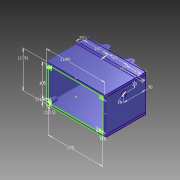
# Autodesk Inventor part: BoxSolidWalls
Saved by Autodesk Inventor 2015 (Build 190159000, 159)
## iProperties
Created: 2015-04-29
Part Number: BoxSolidWalls
Material: ABS Plastic
Document SubType Name: Modeling
Designer: Akovo_000
Mass: 583.352 g
Surface Area: 1681.04 cm^2
Volume: 550.333 cm^3
Density: 1.06 g/cm^3
Appearance: Smooth - White
Author: Akovo_000
Autodesk Inventor part; units mm, degrees
note: some values were not read from the file. Chosen so that the rebuilt part matches the saved one: sketch regions of "LensplateMount".
(part 1 of 2)
ref_plane "YZ Plane" through (0, 0, 0) normal (1, 0, 0) x (0, 1, 0)
ref_plane "XZ Plane" through (0, 0, 0) normal (0, 1, 0) x (-1, 0, 0)
ref_plane "XY Plane" through (0, 0, 0) normal (0, 0, 1) x (1, 0, 0)
sketch "BasicBox" plane through (0, 0, 0) normal (0, 1, 0) x (-1, 0, 0)
  line L0 (88.0422, 45.0444) -> (-86.9578, 45.0444)
  line L1 (-86.9578, 45.0444) -> (-86.9578, -59.9556)
  line L2 (-86.9578, -59.9556) -> (88.0422, -59.9556)
  line L3 (88.0422, -59.9556) -> (88.0422, 45.0444)
  line L4 (95.0422, 52.0444) -> (-93.9578, 52.0444)
  line L5 (-93.9578, 52.0444) -> (-93.9578, -66.9556)
  line L6 (-93.9578, -66.9556) -> (95.0422, -66.9556)
  line L7 (95.0422, -66.9556) -> (95.0422, 52.0444)
  line L8 (88.0422, 45.0444) -> (88.0422, 45.5444) construction
  line L9 (88.0422, 45.0444) -> (88.5422, 45.0444) construction
  line L10 (88.0422, -59.9556) -> (88.0422, -60.4556) construction
  line L11 (88.0422, -59.9556) -> (88.5422, -59.9556) construction
  line L12 (-86.9578, -59.9556) -> (-86.9578, -60.4556) construction
  line L13 (-86.9578, 45.0444) -> (-86.9578, 45.5444) construction
  line L14 (-86.9578, 45.0444) -> (-87.4578, 45.0444) construction
  line L15 (-86.9578, -59.9556) -> (-87.4578, -59.9556) construction
  line L16 (-87.4578, -60.4556) -> (-87.4578, -59.9556)
  line L17 (-87.4578, 45.5444) -> (-86.9578, 45.5444)
  line L18 (88.5422, 45.5444) -> (88.5422, -59.9556)
  line L19 (88.5422, -60.4556) -> (88.0422, -60.4556)
  line L20 (88.5422, 45.0444) -> (95.0422, 45.0444) construction
  line L21 (88.0422, 45.5444) -> (88.0422, 52.0444) construction
  line L22 (-86.9578, 45.5444) -> (88.5422, 45.5444)
  line L23 (-87.4578, 45.0444) -> (-87.4578, 45.5444)
  line L24 (-87.4578, -59.9556) -> (-87.4578, 45.0444)
  line L25 (-86.9578, -60.4556) -> (-87.4578, -60.4556)
  line L26 (88.5422, -59.9556) -> (88.5422, -60.4556)
  line L27 (88.0422, -60.4556) -> (-86.9578, -60.4556)
  line L28 (88.5422, -59.9556) -> (95.0422, -59.9556) construction
  line L29 (88.0422, -60.4556) -> (88.0422, -66.9556) construction
  line L30 (-87.4578, 45.0444) -> (-93.9578, 45.0444) construction
  line L31 (-86.9578, 45.5444) -> (-86.9578, 52.0444) construction
  line L32 (-87.4578, -59.9556) -> (-93.9578, -59.9556) construction
  line L33 (-86.9578, -60.4556) -> (-86.9578, -66.9556) construction
  line L34 (-76.9578, -59.9556) -> (-76.9578, -49.9556)
  line L35 (-76.9578, -49.9556) -> (-86.9578, -49.9556)
  line L36 (-76.9578, 45.0444) -> (-76.9578, 35.0444)
  line L37 (-76.9578, 35.0444) -> (-86.9578, 35.0444)
  line L38 (78.5422, 45.0444) -> (78.5422, 35.0444)
  line L39 (78.5422, 35.0444) -> (88.0422, 35.0444)
  line L40 (88.5422, -49.9556) -> (78.5422, -49.9556)
  line L41 (78.5422, -49.9556) -> (78.5422, -59.9556)
  line L42 (78.5422, 45.0444) -> (78.5422, 52.0444)
  line L43 (88.0422, 35.0444) -> (95.0422, 35.0444)
  line L44 (78.5422, -59.9556) -> (78.5422, -66.9556)
  line L45 (88.5422, -49.9556) -> (95.0422, -49.9556)
  line L46 (-80.8956, -52.9556) -> (-78.8749, -56.4556)
  line L47 (-78.8749, -56.4556) -> (-80.8956, -59.9556)
  line L48 (-80.8956, -59.9556) -> (-84.9371, -59.9556)
  line L49 (-84.9371, -59.9556) -> (-86.9578, -56.4556)
  line L50 (-86.9578, -56.4556) -> (-84.9371, -52.9556)
  line L51 (-84.9371, -52.9556) -> (-80.8956, -52.9556)
  line L52 (-80.8956, 45.0444) -> (-78.8749, 41.5444)
  line L53 (-78.8749, 41.5444) -> (-80.8956, 38.0444)
  line L54 (-80.8956, 38.0444) -> (-84.9371, 38.0444)
  line L55 (-84.9371, 38.0444) -> (-86.9578, 41.5444)
  line L56 (-86.9578, 41.5444) -> (-84.9371, 45.0444)
  line L57 (-84.9371, 45.0444) -> (-80.8956, 45.0444)
  line L58 (86.0215, 45.0444) -> (88.0422, 41.5444)
  line L59 (88.0422, 41.5444) -> (86.0215, 38.0444)
  line L60 (86.0215, 38.0444) -> (81.98, 38.0444)
  line L61 (81.98, 38.0444) -> (79.9593, 41.5444)
  line L62 (79.9593, 41.5444) -> (81.98, 45.0444)
  line L63 (81.98, 45.0444) -> (86.0215, 45.0444)
  line L64 (86.0215, -52.9556) -> (88.0422, -56.4556)
  line L65 (88.0422, -56.4556) -> (86.0215, -59.9556)
  line L66 (86.0215, -59.9556) -> (81.98, -59.9556)
  line L67 (81.98, -59.9556) -> (79.9593, -56.4556)
  line L68 (79.9593, -56.4556) -> (81.98, -52.9556)
  line L69 (81.98, -52.9556) -> (86.0215, -52.9556)
  circle A0 centre (84.0007, 41.5444) radius 2
  circle A1 centre (84.0007, -56.4556) radius 2
  circle A2 centre (-82.9163, -56.4556) radius 2
  circle A3 centre (-82.9163, 41.5444) radius 2
  point P0 (0, 0)
  dimension "d2" = 105
  dimension "d3" = 175
  dimension "d4" = 7
  dimension "d68" = 0.5
  dimension "d71" = 7
  dimension "d94" = 10
  dimension "d95" = 189
  dimension "d96" = 119
  dimension "d97" = 7
  dimension "d98" = 0
  dimension "d101" = 0
  dimension "d102" = 4
  dimension "d105" = 0
  dimension "d106" = 0
  dimension "d109" = 10.5
  dimension "d110" = 11.0414
  constraints: 140 end point, 29 point on line, 22 perpendicular, 14 equal length, 9 parallel, 6 vertical, 5 collinear, 4 centre point, 4 coincident, 4 horizontal, 3 equal radius, 52 other
  measures "d2" distance of L28.end L20.end
  measures "d3" distance of L29.end L33.end
  measures "d4" distance of L6.end L28.end
  measures "d68" distance of L16.start L12.end
  measures "d71" distance of L6.end L29.end
  measures "d94" distance of L34.start L34.end
  measures "d95" distance between parallel lines of L7 L5
  measures "d96" distance between parallel lines of L4 L6
  measures "d97" distance between parallel lines of L51 L48
  measures "d98" distance from line of L1 L49.end
  measures "d101" distance from line of L3 L64.end
  measures "d102" diameter of A0
  measures "d105" distance from line of L1 L55.end
  measures "d106" distance from line of L3 L58.end
  measures "d109" distance from line of L6 point (84.001, -56.456)
  measures "d110" distance from line of L7 point (84.001, -56.456)
extrude "Extrusion1" add sketch "BasicBox" along normal blind 131 contours L0 L42 L22 L18 L43 L3 | L43 L18 L40 L3 | L0 L1 L2 L44 L27 L25 L16 L24 L23 L17 L22 L42 | L40 L18 L26 L19 L27 L44 L2 L3 | L43 L7 L45 L18 | L18 L22 L42 L4 L7 L43 | L22 L17 L23 L24 L16 L25 L27 L44 L6 L5 L4 L42 | L45 L7 L6 L44 L27 L19 L26 L18
sketch "LongerHonycomb" plane through (-95.0422, 0, 52.0444) normal (0, 0, 1) x (1, 0, 0)
  line L0 (0, 131) -> (189, 131)
  line L1 (189, 131) -> (189, 0)
  line L2 (189, 0) -> (0, 0)
  line L3 (0, 0) -> (0, 131)
  line L4 (0, 131) -> (189, 131) projected
  line L5 (182, 131) -> (182, 0)
  line L6 (7, 131) -> (7, 0)
  line L7 (182, 131) -> (7, 131) projected
  line L8 (7, 0) -> (182, 0) projected
  line L9 (21.2583, 115) -> (13.7528, 115)
  line L10 (13.7528, 115) -> (10, 121.5)
  line L11 (10, 121.5) -> (13.7528, 128)
  line L12 (13.7528, 128) -> (21.2583, 128)
  line L13 (21.2583, 128) -> (25.0111, 121.5)
  line L14 (25.0111, 121.5) -> (21.2583, 115)
  line L15 (36.8468, 114) -> (33.094, 107.5)
  line L16 (33.094, 107.5) -> (25.5885, 107.5)
  line L17 (25.5885, 107.5) -> (21.8357, 114)
  line L18 (21.8357, 114) -> (25.5885, 120.5)
  line L19 (25.5885, 120.5) -> (33.094, 120.5)
  line L20 (33.094, 120.5) -> (36.8468, 114)
  line L21 (44.9583, 115) -> (37.4528, 115)
  line L22 (37.4528, 115) -> (33.7, 121.5)
  line L23 (33.7, 121.5) -> (37.4528, 128)
  line L24 (37.4528, 128) -> (44.9583, 128)
  line L25 (44.9583, 128) -> (48.7111, 121.5)
  line L26 (48.7111, 121.5) -> (44.9583, 115)
  line L27 (60.5468, 114) -> (56.794, 107.5)
  line L28 (56.794, 107.5) -> (49.2885, 107.5)
  line L29 (49.2885, 107.5) -> (45.5357, 114)
  line L30 (45.5357, 114) -> (49.2885, 120.5)
  line L31 (49.2885, 120.5) -> (56.794, 120.5)
  line L32 (56.794, 120.5) -> (60.5468, 114)
  line L33 (68.6583, 115) -> (61.1528, 115)
  line L34 (61.1528, 115) -> (57.4, 121.5)
  line L35 (57.4, 121.5) -> (61.1528, 128)
  line L36 (61.1528, 128) -> (68.6583, 128)
  line L37 (68.6583, 128) -> (72.4111, 121.5)
  line L38 (72.4111, 121.5) -> (68.6583, 115)
  line L39 (84.2468, 114) -> (80.494, 107.5)
  line L40 (80.494, 107.5) -> (72.9885, 107.5)
  line L41 (72.9885, 107.5) -> (69.2357, 114)
  line L42 (69.2357, 114) -> (72.9885, 120.5)
  line L43 (72.9885, 120.5) -> (80.494, 120.5)
  line L44 (80.494, 120.5) -> (84.2468, 114)
  line L45 (92.3583, 115) -> (84.8528, 115)
  line L46 (84.8528, 115) -> (81.1, 121.5)
  line L47 (81.1, 121.5) -> (84.8528, 128)
  line L48 (84.8528, 128) -> (92.3583, 128)
  line L49 (92.3583, 128) -> (96.1111, 121.5)
  line L50 (96.1111, 121.5) -> (92.3583, 115)
  line L51 (107.9468, 114) -> (104.194, 107.5)
  line L52 (104.194, 107.5) -> (96.6885, 107.5)
  line L53 (96.6885, 107.5) -> (92.9357, 114)
  line L54 (92.9357, 114) -> (96.6885, 120.5)
  line L55 (96.6885, 120.5) -> (104.194, 120.5)
  line L56 (104.194, 120.5) -> (107.9468, 114)
  line L57 (116.0583, 115) -> (108.5528, 115)
  line L58 (108.5528, 115) -> (104.8, 121.5)
  line L59 (104.8, 121.5) -> (108.5528, 128)
  line L60 (108.5528, 128) -> (116.0583, 128)
  line L61 (116.0583, 128) -> (119.8111, 121.5)
  line L62 (119.8111, 121.5) -> (116.0583, 115)
  line L63 (131.6468, 114) -> (127.894, 107.5)
  line L64 (127.894, 107.5) -> (120.3885, 107.5)
  line L65 (120.3885, 107.5) -> (116.6357, 114)
  line L66 (116.6357, 114) -> (120.3885, 120.5)
  line L67 (120.3885, 120.5) -> (127.894, 120.5)
  line L68 (127.894, 120.5) -> (131.6468, 114)
  line L69 (139.7583, 115) -> (132.2528, 115)
  line L70 (132.2528, 115) -> (128.5, 121.5)
  line L71 (128.5, 121.5) -> (132.2528, 128)
  line L72 (132.2528, 128) -> (139.7583, 128)
  line L73 (139.7583, 128) -> (143.5111, 121.5)
  line L74 (143.5111, 121.5) -> (139.7583, 115)
  line L75 (155.3468, 114) -> (151.594, 107.5)
  line L76 (151.594, 107.5) -> (144.0885, 107.5)
  line L77 (144.0885, 107.5) -> (140.3357, 114)
  line L78 (140.3357, 114) -> (144.0885, 120.5)
  line L79 (144.0885, 120.5) -> (151.594, 120.5)
  line L80 (151.594, 120.5) -> (155.3468, 114)
  line L81 (21.2583, 100) -> (13.7528, 100)
  line L82 (13.7528, 100) -> (10, 106.5)
  line L83 (10, 106.5) -> (13.7528, 113)
  line L84 (13.7528, 113) -> (21.2583, 113)
  line L85 (21.2583, 113) -> (25.0111, 106.5)
  line L86 (25.0111, 106.5) -> (21.2583, 100)
  line L87 (36.8468, 99) -> (33.094, 92.5)
  line L88 (33.094, 92.5) -> (25.5885, 92.5)
  line L89 (25.5885, 92.5) -> (21.8357, 99)
  line L90 (21.8357, 99) -> (25.5885, 105.5)
  line L91 (25.5885, 105.5) -> (33.094, 105.5)
  line L92 (33.094, 105.5) -> (36.8468, 99)
  line L93 (44.9583, 100) -> (37.4528, 100)
  line L94 (37.4528, 100) -> (33.7, 106.5)
  line L95 (33.7, 106.5) -> (37.4528, 113)
  line L96 (37.4528, 113) -> (44.9583, 113)
  line L97 (44.9583, 113) -> (48.7111, 106.5)
  line L98 (48.7111, 106.5) -> (44.9583, 100)
  line L99 (60.5468, 99) -> (56.794, 92.5)
  line L100 (56.794, 92.5) -> (49.2885, 92.5)
  line L101 (49.2885, 92.5) -> (45.5357, 99)
  line L102 (45.5357, 99) -> (49.2885, 105.5)
  line L103 (49.2885, 105.5) -> (56.794, 105.5)
  line L104 (56.794, 105.5) -> (60.5468, 99)
  line L105 (68.6583, 100) -> (61.1528, 100)
  line L106 (61.1528, 100) -> (57.4, 106.5)
  line L107 (57.4, 106.5) -> (61.1528, 113)
  line L108 (61.1528, 113) -> (68.6583, 113)
  line L109 (68.6583, 113) -> (72.4111, 106.5)
  line L110 (72.4111, 106.5) -> (68.6583, 100)
  line L111 (84.2468, 99) -> (80.494, 92.5)
  line L112 (80.494, 92.5) -> (72.9885, 92.5)
  line L113 (72.9885, 92.5) -> (69.2357, 99)
  line L114 (69.2357, 99) -> (72.9885, 105.5)
  line L115 (72.9885, 105.5) -> (80.494, 105.5)
  line L116 (80.494, 105.5) -> (84.2468, 99)
  line L117 (92.3583, 100) -> (84.8528, 100)
  line L118 (84.8528, 100) -> (81.1, 106.5)
  line L119 (81.1, 106.5) -> (84.8528, 113)
  line L120 (84.8528, 113) -> (92.3583, 113)
  line L121 (92.3583, 113) -> (96.1111, 106.5)
  line L122 (96.1111, 106.5) -> (92.3583, 100)
  line L123 (107.9468, 99) -> (104.194, 92.5)
  line L124 (104.194, 92.5) -> (96.6885, 92.5)
  line L125 (96.6885, 92.5) -> (92.9357, 99)
  line L126 (92.9357, 99) -> (96.6885, 105.5)
  line L127 (96.6885, 105.5) -> (104.194, 105.5)
  line L128 (104.194, 105.5) -> (107.9468, 99)
  line L129 (116.0583, 100) -> (108.5528, 100)
  line L130 (108.5528, 100) -> (104.8, 106.5)
  line L131 (104.8, 106.5) -> (108.5528, 113)
  line L132 (108.5528, 113) -> (116.0583, 113)
  line L133 (116.0583, 113) -> (119.8111, 106.5)
  line L134 (119.8111, 106.5) -> (116.0583, 100)
  line L135 (131.6468, 99) -> (127.894, 92.5)
  line L136 (127.894, 92.5) -> (120.3885, 92.5)
  line L137 (120.3885, 92.5) -> (116.6357, 99)
  line L138 (116.6357, 99) -> (120.3885, 105.5)
  line L139 (120.3885, 105.5) -> (127.894, 105.5)
  line L140 (127.894, 105.5) -> (131.6468, 99)
  line L141 (139.7583, 100) -> (132.2528, 100)
  line L142 (132.2528, 100) -> (128.5, 106.5)
  line L143 (128.5, 106.5) -> (132.2528, 113)
  line L144 (132.2528, 113) -> (139.7583, 113)
  line L145 (139.7583, 113) -> (143.5111, 106.5)
  line L146 (143.5111, 106.5) -> (139.7583, 100)
  line L147 (155.3468, 99) -> (151.594, 92.5)
  line L148 (151.594, 92.5) -> (144.0885, 92.5)
  line L149 (144.0885, 92.5) -> (140.3357, 99)
  line L150 (140.3357, 99) -> (144.0885, 105.5)
  line L151 (144.0885, 105.5) -> (151.594, 105.5)
  line L152 (151.594, 105.5) -> (155.3468, 99)
  line L153 (21.2583, 85) -> (13.7528, 85)
  line L154 (13.7528, 85) -> (10, 91.5)
  line L155 (10, 91.5) -> (13.7528, 98)
  line L156 (13.7528, 98) -> (21.2583, 98)
  line L157 (21.2583, 98) -> (25.0111, 91.5)
  line L158 (25.0111, 91.5) -> (21.2583, 85)
  line L159 (36.8468, 84) -> (33.094, 77.5)
  line L160 (33.094, 77.5) -> (25.5885, 77.5)
  line L161 (25.5885, 77.5) -> (21.8357, 84)
  line L162 (21.8357, 84) -> (25.5885, 90.5)
  line L163 (25.5885, 90.5) -> (33.094, 90.5)
  line L164 (33.094, 90.5) -> (36.8468, 84)
  line L165 (44.9583, 85) -> (37.4528, 85)
  line L166 (37.4528, 85) -> (33.7, 91.5)
  line L167 (33.7, 91.5) -> (37.4528, 98)
  line L168 (37.4528, 98) -> (44.9583, 98)
  line L169 (44.9583, 98) -> (48.7111, 91.5)
  line L170 (48.7111, 91.5) -> (44.9583, 85)
  line L171 (60.5468, 84) -> (56.794, 77.5)
  line L172 (56.794, 77.5) -> (49.2885, 77.5)
  line L173 (49.2885, 77.5) -> (45.5357, 84)
  line L174 (45.5357, 84) -> (49.2885, 90.5)
  line L175 (49.2885, 90.5) -> (56.794, 90.5)
  line L176 (56.794, 90.5) -> (60.5468, 84)
  line L177 (68.6583, 85) -> (61.1528, 85)
  line L178 (61.1528, 85) -> (57.4, 91.5)
  line L179 (57.4, 91.5) -> (61.1528, 98)
  line L180 (61.1528, 98) -> (68.6583, 98)
  line L181 (68.6583, 98) -> (72.4111, 91.5)
  line L182 (72.4111, 91.5) -> (68.6583, 85)
  line L183 (84.2468, 84) -> (80.494, 77.5)
  line L184 (80.494, 77.5) -> (72.9885, 77.5)
  line L185 (72.9885, 77.5) -> (69.2357, 84)
  line L186 (69.2357, 84) -> (72.9885, 90.5)
  line L187 (72.9885, 90.5) -> (80.494, 90.5)
  line L188 (80.494, 90.5) -> (84.2468, 84)
  line L189 (92.3583, 85) -> (84.8528, 85)
  line L190 (84.8528, 85) -> (81.1, 91.5)
  line L191 (81.1, 91.5) -> (84.8528, 98)
  line L192 (84.8528, 98) -> (92.3583, 98)
  line L193 (92.3583, 98) -> (96.1111, 91.5)
  line L194 (96.1111, 91.5) -> (92.3583, 85)
  line L195 (107.9468, 84) -> (104.194, 77.5)
  line L196 (104.194, 77.5) -> (96.6885, 77.5)
  line L197 (96.6885, 77.5) -> (92.9357, 84)
  line L198 (92.9357, 84) -> (96.6885, 90.5)
  line L199 (96.6885, 90.5) -> (104.194, 90.5)
  line L200 (104.194, 90.5) -> (107.9468, 84)
  line L201 (116.0583, 85) -> (108.5528, 85)
  line L202 (108.5528, 85) -> (104.8, 91.5)
  line L203 (104.8, 91.5) -> (108.5528, 98)
  line L204 (108.5528, 98) -> (116.0583, 98)
  line L205 (116.0583, 98) -> (119.8111, 91.5)
  line L206 (119.8111, 91.5) -> (116.0583, 85)
  line L207 (131.6468, 84) -> (127.894, 77.5)
  line L208 (127.894, 77.5) -> (120.3885, 77.5)
  line L209 (120.3885, 77.5) -> (116.6357, 84)
  line L210 (116.6357, 84) -> (120.3885, 90.5)
  line L211 (120.3885, 90.5) -> (127.894, 90.5)
  line L212 (127.894, 90.5) -> (131.6468, 84)
  line L213 (139.7583, 85) -> (132.2528, 85)
  line L214 (132.2528, 85) -> (128.5, 91.5)
  line L215 (128.5, 91.5) -> (132.2528, 98)
  line L216 (132.2528, 98) -> (139.7583, 98)
  line L217 (139.7583, 98) -> (143.5111, 91.5)
  line L218 (143.5111, 91.5) -> (139.7583, 85)
  line L219 (155.3468, 84) -> (151.594, 77.5)
  line L220 (151.594, 77.5) -> (144.0885, 77.5)
  line L221 (144.0885, 77.5) -> (140.3357, 84)
  line L222 (140.3357, 84) -> (144.0885, 90.5)
  line L223 (144.0885, 90.5) -> (151.594, 90.5)
  line L224 (151.594, 90.5) -> (155.3468, 84)
  line L225 (21.2583, 70) -> (13.7528, 70)
  line L226 (13.7528, 70) -> (10, 76.5)
  line L227 (10, 76.5) -> (13.7528, 83)
  line L228 (13.7528, 83) -> (21.2583, 83)
  line L229 (21.2583, 83) -> (25.0111, 76.5)
  line L230 (25.0111, 76.5) -> (21.2583, 70)
  line L231 (36.8468, 69) -> (33.094, 62.5)
  line L232 (33.094, 62.5) -> (25.5885, 62.5)
  line L233 (25.5885, 62.5) -> (21.8357, 69)
  line L234 (21.8357, 69) -> (25.5885, 75.5)
  line L235 (25.5885, 75.5) -> (33.094, 75.5)
  line L236 (33.094, 75.5) -> (36.8468, 69)
  line L237 (44.9583, 70) -> (37.4528, 70)
  line L238 (37.4528, 70) -> (33.7, 76.5)
  line L239 (33.7, 76.5) -> (37.4528, 83)
  line L240 (37.4528, 83) -> (44.9583, 83)
  line L241 (44.9583, 83) -> (48.7111, 76.5)
  line L242 (48.7111, 76.5) -> (44.9583, 70)
  line L243 (60.5468, 69) -> (56.794, 62.5)
  line L244 (56.794, 62.5) -> (49.2885, 62.5)
  line L245 (49.2885, 62.5) -> (45.5357, 69)
  line L246 (45.5357, 69) -> (49.2885, 75.5)
  line L247 (49.2885, 75.5) -> (56.794, 75.5)
  line L248 (56.794, 75.5) -> (60.5468, 69)
  line L249 (68.6583, 70) -> (61.1528, 70)
  line L250 (61.1528, 70) -> (57.4, 76.5)
  line L251 (57.4, 76.5) -> (61.1528, 83)
  line L252 (61.1528, 83) -> (68.6583, 83)
  line L253 (68.6583, 83) -> (72.4111, 76.5)
  line L254 (72.4111, 76.5) -> (68.6583, 70)
  line L255 (84.2468, 69) -> (80.494, 62.5)
  line L256 (80.494, 62.5) -> (72.9885, 62.5)
  line L257 (72.9885, 62.5) -> (69.2357, 69)
  line L258 (69.2357, 69) -> (72.9885, 75.5)
  line L259 (72.9885, 75.5) -> (80.494, 75.5)
  line L260 (80.494, 75.5) -> (84.2468, 69)
  line L261 (92.3583, 70) -> (84.8528, 70)
  line L262 (84.8528, 70) -> (81.1, 76.5)
  line L263 (81.1, 76.5) -> (84.8528, 83)
  line L264 (84.8528, 83) -> (92.3583, 83)
  line L265 (92.3583, 83) -> (96.1111, 76.5)
  line L266 (96.1111, 76.5) -> (92.3583, 70)
  line L267 (107.9468, 69) -> (104.194, 62.5)
  line L268 (104.194, 62.5) -> (96.6885, 62.5)
  line L269 (96.6885, 62.5) -> (92.9357, 69)
  line L270 (92.9357, 69) -> (96.6885, 75.5)
  line L271 (96.6885, 75.5) -> (104.194, 75.5)
  line L272 (104.194, 75.5) -> (107.9468, 69)
  line L273 (116.0583, 70) -> (108.5528, 70)
  line L274 (108.5528, 70) -> (104.8, 76.5)
  line L275 (104.8, 76.5) -> (108.5528, 83)
  line L276 (108.5528, 83) -> (116.0583, 83)
  line L277 (116.0583, 83) -> (119.8111, 76.5)
  line L278 (119.8111, 76.5) -> (116.0583, 70)
  line L279 (131.6468, 69) -> (127.894, 62.5)
  line L280 (127.894, 62.5) -> (120.3885, 62.5)
  line L281 (120.3885, 62.5) -> (116.6357, 69)
  line L282 (116.6357, 69) -> (120.3885, 75.5)
  line L283 (120.3885, 75.5) -> (127.894, 75.5)
  line L284 (127.894, 75.5) -> (131.6468, 69)
  line L285 (139.7583, 70) -> (132.2528, 70)
  line L286 (132.2528, 70) -> (128.5, 76.5)
  line L287 (128.5, 76.5) -> (132.2528, 83)
  line L288 (132.2528, 83) -> (139.7583, 83)
  line L289 (139.7583, 83) -> (143.5111, 76.5)
  line L290 (143.5111, 76.5) -> (139.7583, 70)
  line L291 (155.3468, 69) -> (151.594, 62.5)
  line L292 (151.594, 62.5) -> (144.0885, 62.5)
  line L293 (144.0885, 62.5) -> (140.3357, 69)
  line L294 (140.3357, 69) -> (144.0885, 75.5)
  line L295 (144.0885, 75.5) -> (151.594, 75.5)
  line L296 (151.594, 75.5) -> (155.3468, 69)
  line L297 (21.2583, 55) -> (13.7528, 55)
  line L298 (13.7528, 55) -> (10, 61.5)
  line L299 (10, 61.5) -> (13.7528, 68)
  line L300 (13.7528, 68) -> (21.2583, 68)
  line L301 (21.2583, 68) -> (25.0111, 61.5)
  line L302 (25.0111, 61.5) -> (21.2583, 55)
  line L303 (36.8468, 54) -> (33.094, 47.5)
  line L304 (33.094, 47.5) -> (25.5885, 47.5)
  line L305 (25.5885, 47.5) -> (21.8357, 54)
  line L306 (21.8357, 54) -> (25.5885, 60.5)
  line L307 (25.5885, 60.5) -> (33.094, 60.5)
  line L308 (33.094, 60.5) -> (36.8468, 54)
  line L309 (44.9583, 55) -> (37.4528, 55)
  line L310 (37.4528, 55) -> (33.7, 61.5)
  line L311 (33.7, 61.5) -> (37.4528, 68)
  line L312 (37.4528, 68) -> (44.9583, 68)
  line L313 (44.9583, 68) -> (48.7111, 61.5)
  line L314 (48.7111, 61.5) -> (44.9583, 55)
  line L315 (60.5468, 54) -> (56.794, 47.5)
  line L316 (56.794, 47.5) -> (49.2885, 47.5)
  line L317 (49.2885, 47.5) -> (45.5357, 54)
  line L318 (45.5357, 54) -> (49.2885, 60.5)
  line L319 (49.2885, 60.5) -> (56.794, 60.5)
  line L320 (56.794, 60.5) -> (60.5468, 54)
  line L321 (68.6583, 55) -> (61.1528, 55)
  line L322 (61.1528, 55) -> (57.4, 61.5)
  line L323 (57.4, 61.5) -> (61.1528, 68)
  line L324 (61.1528, 68) -> (68.6583, 68)
  line L325 (68.6583, 68) -> (72.4111, 61.5)
  line L326 (72.4111, 61.5) -> (68.6583, 55)
  line L327 (84.2468, 54) -> (80.494, 47.5)
  line L328 (80.494, 47.5) -> (72.9885, 47.5)
  line L329 (72.9885, 47.5) -> (69.2357, 54)
  line L330 (69.2357, 54) -> (72.9885, 60.5)
  line L331 (72.9885, 60.5) -> (80.494, 60.5)
  line L332 (80.494, 60.5) -> (84.2468, 54)
  line L333 (92.3583, 55) -> (84.8528, 55)
  line L334 (84.8528, 55) -> (81.1, 61.5)
  line L335 (81.1, 61.5) -> (84.8528, 68)
  line L336 (84.8528, 68) -> (92.3583, 68)
  line L337 (92.3583, 68) -> (96.1111, 61.5)
  line L338 (96.1111, 61.5) -> (92.3583, 55)
  line L339 (107.9468, 54) -> (104.194, 47.5)
  line L340 (104.194, 47.5) -> (96.6885, 47.5)
  line L341 (96.6885, 47.5) -> (92.9357, 54)
  line L342 (92.9357, 54) -> (96.6885, 60.5)
  line L343 (96.6885, 60.5) -> (104.194, 60.5)
  line L344 (104.194, 60.5) -> (107.9468, 54)
  line L345 (116.0583, 55) -> (108.5528, 55)
  line L346 (108.5528, 55) -> (104.8, 61.5)
  line L347 (104.8, 61.5) -> (108.5528, 68)
  line L348 (108.5528, 68) -> (116.0583, 68)
  line L349 (116.0583, 68) -> (119.8111, 61.5)
  line L350 (119.8111, 61.5) -> (116.0583, 55)
  line L351 (131.6468, 54) -> (127.894, 47.5)
  line L352 (127.894, 47.5) -> (120.3885, 47.5)
  line L353 (120.3885, 47.5) -> (116.6357, 54)
  line L354 (116.6357, 54) -> (120.3885, 60.5)
  line L355 (120.3885, 60.5) -> (127.894, 60.5)
  line L356 (127.894, 60.5) -> (131.6468, 54)
  line L357 (139.7583, 55) -> (132.2528, 55)
  line L358 (132.2528, 55) -> (128.5, 61.5)
  line L359 (128.5, 61.5) -> (132.2528, 68)
  line L360 (132.2528, 68) -> (139.7583, 68)
  line L361 (139.7583, 68) -> (143.5111, 61.5)
  line L362 (143.5111, 61.5) -> (139.7583, 55)
  line L363 (155.3468, 54) -> (151.594, 47.5)
  line L364 (151.594, 47.5) -> (144.0885, 47.5)
  line L365 (144.0885, 47.5) -> (140.3357, 54)
  line L366 (140.3357, 54) -> (144.0885, 60.5)
  line L367 (144.0885, 60.5) -> (151.594, 60.5)
  line L368 (151.594, 60.5) -> (155.3468, 54)
  line L369 (21.2583, 40) -> (13.7528, 40)
  line L370 (13.7528, 40) -> (10, 46.5)
  line L371 (10, 46.5) -> (13.7528, 53)
  line L372 (13.7528, 53) -> (21.2583, 53)
  line L373 (21.2583, 53) -> (25.0111, 46.5)
  line L374 (25.0111, 46.5) -> (21.2583, 40)
  line L375 (36.8468, 39) -> (33.094, 32.5)
  line L376 (33.094, 32.5) -> (25.5885, 32.5)
  line L377 (25.5885, 32.5) -> (21.8357, 39)
  line L378 (21.8357, 39) -> (25.5885, 45.5)
  line L379 (25.5885, 45.5) -> (33.094, 45.5)
  line L380 (33.094, 45.5) -> (36.8468, 39)
  line L381 (44.9583, 40) -> (37.4528, 40)
  line L382 (37.4528, 40) -> (33.7, 46.5)
  line L383 (33.7, 46.5) -> (37.4528, 53)
  line L384 (37.4528, 53) -> (44.9583, 53)
  line L385 (44.9583, 53) -> (48.7111, 46.5)
  line L386 (48.7111, 46.5) -> (44.9583, 40)
  line L387 (60.5468, 39) -> (56.794, 32.5)
  line L388 (56.794, 32.5) -> (49.2885, 32.5)
  line L389 (49.2885, 32.5) -> (45.5357, 39)
  line L390 (45.5357, 39) -> (49.2885, 45.5)
  line L391 (49.2885, 45.5) -> (56.794, 45.5)
  line L392 (56.794, 45.5) -> (60.5468, 39)
  line L393 (68.6583, 40) -> (61.1528, 40)
  line L394 (61.1528, 40) -> (57.4, 46.5)
  line L395 (57.4, 46.5) -> (61.1528, 53)
  line L396 (61.1528, 53) -> (68.6583, 53)
  line L397 (68.6583, 53) -> (72.4111, 46.5)
  line L398 (72.4111, 46.5) -> (68.6583, 40)
  line L399 (84.2468, 39) -> (80.494, 32.5)
  line L400 (80.494, 32.5) -> (72.9885, 32.5)
  line L401 (72.9885, 32.5) -> (69.2357, 39)
  line L402 (69.2357, 39) -> (72.9885, 45.5)
  line L403 (72.9885, 45.5) -> (80.494, 45.5)
  line L404 (80.494, 45.5) -> (84.2468, 39)
  line L405 (92.3583, 40) -> (84.8528, 40)
  line L406 (84.8528, 40) -> (81.1, 46.5)
  line L407 (81.1, 46.5) -> (84.8528, 53)
  line L408 (84.8528, 53) -> (92.3583, 53)
  line L409 (92.3583, 53) -> (96.1111, 46.5)
  line L410 (96.1111, 46.5) -> (92.3583, 40)
  line L411 (107.9468, 39) -> (104.194, 32.5)
  line L412 (104.194, 32.5) -> (96.6885, 32.5)
  line L413 (96.6885, 32.5) -> (92.9357, 39)
  line L414 (92.9357, 39) -> (96.6885, 45.5)
  line L415 (96.6885, 45.5) -> (104.194, 45.5)
  line L416 (104.194, 45.5) -> (107.9468, 39)
  line L417 (116.0583, 40) -> (108.5528, 40)
  line L418 (108.5528, 40) -> (104.8, 46.5)
  line L419 (104.8, 46.5) -> (108.5528, 53)
  line L420 (108.5528, 53) -> (116.0583, 53)
  line L421 (116.0583, 53) -> (119.8111, 46.5)
  line L422 (119.8111, 46.5) -> (116.0583, 40)
  line L423 (131.6468, 39) -> (127.894, 32.5)
  line L424 (127.894, 32.5) -> (120.3885, 32.5)
  line L425 (120.3885, 32.5) -> (116.6357, 39)
  line L426 (116.6357, 39) -> (120.3885, 45.5)
  line L427 (120.3885, 45.5) -> (127.894, 45.5)
  line L428 (127.894, 45.5) -> (131.6468, 39)
  line L429 (139.7583, 40) -> (132.2528, 40)
  line L430 (132.2528, 40) -> (128.5, 46.5)
  line L431 (128.5, 46.5) -> (132.2528, 53)
  line L432 (132.2528, 53) -> (139.7583, 53)
  line L433 (139.7583, 53) -> (143.5111, 46.5)
  line L434 (143.5111, 46.5) -> (139.7583, 40)
  line L435 (155.3468, 39) -> (151.594, 32.5)
  line L436 (151.594, 32.5) -> (144.0885, 32.5)
  line L437 (144.0885, 32.5) -> (140.3357, 39)
  line L438 (140.3357, 39) -> (144.0885, 45.5)
  line L439 (144.0885, 45.5) -> (151.594, 45.5)
  line L440 (151.594, 45.5) -> (155.3468, 39)
  line L441 (21.2583, 25) -> (13.7528, 25)
  line L442 (13.7528, 25) -> (10, 31.5)
  line L443 (10, 31.5) -> (13.7528, 38)
  line L444 (13.7528, 38) -> (21.2583, 38)
  line L445 (21.2583, 38) -> (25.0111, 31.5)
  line L446 (25.0111, 31.5) -> (21.2583, 25)
  line L447 (36.8468, 24) -> (33.094, 17.5)
  line L448 (33.094, 17.5) -> (25.5885, 17.5)
  line L449 (25.5885, 17.5) -> (21.8357, 24)
  line L450 (21.8357, 24) -> (25.5885, 30.5)
  line L451 (25.5885, 30.5) -> (33.094, 30.5)
  line L452 (33.094, 30.5) -> (36.8468, 24)
  line L453 (44.9583, 25) -> (37.4528, 25)
  line L454 (37.4528, 25) -> (33.7, 31.5)
  line L455 (33.7, 31.5) -> (37.4528, 38)
  line L456 (37.4528, 38) -> (44.9583, 38)
  line L457 (44.9583, 38) -> (48.7111, 31.5)
  line L458 (48.7111, 31.5) -> (44.9583, 25)
  line L459 (60.5468, 24) -> (56.794, 17.5)
  line L460 (56.794, 17.5) -> (49.2885, 17.5)
  line L461 (49.2885, 17.5) -> (45.5357, 24)
  line L462 (45.5357, 24) -> (49.2885, 30.5)
  line L463 (49.2885, 30.5) -> (56.794, 30.5)
  line L464 (56.794, 30.5) -> (60.5468, 24)
  line L465 (68.6583, 25) -> (61.1528, 25)
  line L466 (61.1528, 25) -> (57.4, 31.5)
  line L467 (57.4, 31.5) -> (61.1528, 38)
  line L468 (61.1528, 38) -> (68.6583, 38)
  line L469 (68.6583, 38) -> (72.4111, 31.5)
  line L470 (72.4111, 31.5) -> (68.6583, 25)
  line L471 (84.2468, 24) -> (80.494, 17.5)
  line L472 (80.494, 17.5) -> (72.9885, 17.5)
  line L473 (72.9885, 17.5) -> (69.2357, 24)
  line L474 (69.2357, 24) -> (72.9885, 30.5)
  line L475 (72.9885, 30.5) -> (80.494, 30.5)
  line L476 (80.494, 30.5) -> (84.2468, 24)
  line L477 (92.3583, 25) -> (84.8528, 25)
  line L478 (84.8528, 25) -> (81.1, 31.5)
  line L479 (81.1, 31.5) -> (84.8528, 38)
  line L480 (84.8528, 38) -> (92.3583, 38)
  line L481 (92.3583, 38) -> (96.1111, 31.5)
  line L482 (96.1111, 31.5) -> (92.3583, 25)
  line L483 (107.9468, 24) -> (104.194, 17.5)
  line L484 (104.194, 17.5) -> (96.6885, 17.5)
  line L485 (96.6885, 17.5) -> (92.9357, 24)
  line L486 (92.9357, 24) -> (96.6885, 30.5)
  line L487 (96.6885, 30.5) -> (104.194, 30.5)
  line L488 (104.194, 30.5) -> (107.9468, 24)
  line L489 (116.0583, 25) -> (108.5528, 25)
  line L490 (108.5528, 25) -> (104.8, 31.5)
  line L491 (104.8, 31.5) -> (108.5528, 38)
  line L492 (108.5528, 38) -> (116.0583, 38)
  line L493 (116.0583, 38) -> (119.8111, 31.5)
  line L494 (119.8111, 31.5) -> (116.0583, 25)
  line L495 (131.6468, 24) -> (127.894, 17.5)
  line L496 (127.894, 17.5) -> (120.3885, 17.5)
  line L497 (120.3885, 17.5) -> (116.6357, 24)
  line L498 (116.6357, 24) -> (120.3885, 30.5)
  line L499 (120.3885, 30.5) -> (127.894, 30.5)
  line L500 (127.894, 30.5) -> (131.6468, 24)
  line L501 (139.7583, 25) -> (132.2528, 25)
  line L502 (132.2528, 25) -> (128.5, 31.5)
  line L503 (128.5, 31.5) -> (132.2528, 38)
  line L504 (132.2528, 38) -> (139.7583, 38)
  line L505 (139.7583, 38) -> (143.5111, 31.5)
  line L506 (143.5111, 31.5) -> (139.7583, 25)
  line L507 (155.3468, 24) -> (151.594, 17.5)
  line L508 (151.594, 17.5) -> (144.0885, 17.5)
  line L509 (144.0885, 17.5) -> (140.3357, 24)
  line L510 (140.3357, 24) -> (144.0885, 30.5)
  line L511 (144.0885, 30.5) -> (151.594, 30.5)
  line L512 (151.594, 30.5) -> (155.3468, 24)
  line L513 (21.2583, 10) -> (13.7528, 10)
  line L514 (13.7528, 10) -> (10, 16.5)
  line L515 (10, 16.5) -> (13.7528, 23)
  line L516 (13.7528, 23) -> (21.2583, 23)
  line L517 (21.2583, 23) -> (25.0111, 16.5)
  line L518 (25.0111, 16.5) -> (21.2583, 10)
  line L519 (44.9583, 10) -> (37.4528, 10)
  line L520 (37.4528, 10) -> (33.7, 16.5)
  line L521 (33.7, 16.5) -> (37.4528, 23)
  line L522 (37.4528, 23) -> (44.9583, 23)
  line L523 (44.9583, 23) -> (48.7111, 16.5)
  line L524 (48.7111, 16.5) -> (44.9583, 10)
  line L525 (68.6583, 10) -> (61.1528, 10)
  line L526 (61.1528, 10) -> (57.4, 16.5)
  line L527 (57.4, 16.5) -> (61.1528, 23)
  line L528 (61.1528, 23) -> (68.6583, 23)
  line L529 (68.6583, 23) -> (72.4111, 16.5)
  line L530 (72.4111, 16.5) -> (68.6583, 10)
  line L531 (92.3583, 10) -> (84.8528, 10)
  line L532 (84.8528, 10) -> (81.1, 16.5)
  line L533 (81.1, 16.5) -> (84.8528, 23)
  line L534 (84.8528, 23) -> (92.3583, 23)
  line L535 (92.3583, 23) -> (96.1111, 16.5)
  line L536 (96.1111, 16.5) -> (92.3583, 10)
  line L537 (116.0583, 10) -> (108.5528, 10)
  line L538 (108.5528, 10) -> (104.8, 16.5)
  line L539 (104.8, 16.5) -> (108.5528, 23)
  line L540 (108.5528, 23) -> (116.0583, 23)
  line L541 (116.0583, 23) -> (119.8111, 16.5)
  line L542 (119.8111, 16.5) -> (116.0583, 10)
  line L543 (139.7583, 10) -> (132.2528, 10)
  line L544 (132.2528, 10) -> (128.5, 16.5)
  line L545 (128.5, 16.5) -> (132.2528, 23)
  line L546 (132.2528, 23) -> (139.7583, 23)
  line L547 (139.7583, 23) -> (143.5111, 16.5)
  line L548 (143.5111, 16.5) -> (139.7583, 10)
  line L549 (25.0111, 121.5) -> (25.5885, 120.5) construction
  line L550 (162.8583, 115) -> (155.3528, 115)
  line L551 (155.3528, 115) -> (151.6, 121.5)
  line L552 (151.6, 121.5) -> (155.3528, 128)
  line L553 (155.3528, 128) -> (162.8583, 128)
  line L554 (162.8583, 128) -> (166.6111, 121.5)
  line L555 (166.6111, 121.5) -> (162.8583, 115)
  line L556 (163.4357, 114) -> (167.1885, 120.5)
  line L557 (167.1885, 107.5) -> (163.4357, 114)
  line L558 (174.694, 107.5) -> (167.1885, 107.5)
  line L559 (178.4468, 114) -> (174.694, 107.5)
  line L560 (174.694, 120.5) -> (178.4468, 114)
  line L561 (167.1885, 120.5) -> (174.694, 120.5)
  line L562 (162.8583, 100) -> (155.3528, 100)
  line L563 (155.3528, 100) -> (151.6, 106.5)
  line L564 (151.6, 106.5) -> (155.3528, 113)
  line L565 (155.3528, 113) -> (162.8583, 113)
  line L566 (162.8583, 113) -> (166.6111, 106.5)
  line L567 (166.6111, 106.5) -> (162.8583, 100)
  line L568 (163.4357, 99) -> (167.1885, 105.5)
  line L569 (167.1885, 92.5) -> (163.4357, 99)
  line L570 (174.694, 92.5) -> (167.1885, 92.5)
  line L571 (178.4468, 99) -> (174.694, 92.5)
  line L572 (174.694, 105.5) -> (178.4468, 99)
  line L573 (167.1885, 105.5) -> (174.694, 105.5)
  line L574 (162.8583, 85) -> (155.3528, 85)
  line L575 (155.3528, 85) -> (151.6, 91.5)
  line L576 (151.6, 91.5) -> (155.3528, 98)
  line L577 (155.3528, 98) -> (162.8583, 98)
  line L578 (162.8583, 98) -> (166.6111, 91.5)
  line L579 (166.6111, 91.5) -> (162.8583, 85)
  line L580 (163.4357, 84) -> (167.1885, 90.5)
  line L581 (167.1885, 77.5) -> (163.4357, 84)
  line L582 (174.694, 77.5) -> (167.1885, 77.5)
  line L583 (178.4468, 84) -> (174.694, 77.5)
  line L584 (174.694, 90.5) -> (178.4468, 84)
  line L585 (167.1885, 90.5) -> (174.694, 90.5)
  line L586 (162.8583, 70) -> (155.3528, 70)
  line L587 (155.3528, 70) -> (151.6, 76.5)
  line L588 (151.6, 76.5) -> (155.3528, 83)
  line L589 (155.3528, 83) -> (162.8583, 83)
  line L590 (162.8583, 83) -> (166.6111, 76.5)
  line L591 (166.6111, 76.5) -> (162.8583, 70)
  line L592 (163.4357, 69) -> (167.1885, 75.5)
  line L593 (167.1885, 62.5) -> (163.4357, 69)
  line L594 (174.694, 62.5) -> (167.1885, 62.5)
  line L595 (178.4468, 69) -> (174.694, 62.5)
  line L596 (174.694, 75.5) -> (178.4468, 69)
  line L597 (167.1885, 75.5) -> (174.694, 75.5)
  line L598 (162.8583, 55) -> (155.3528, 55)
  line L599 (155.3528, 55) -> (151.6, 61.5)
  line L600 (151.6, 61.5) -> (155.3528, 68)
  line L601 (155.3528, 68) -> (162.8583, 68)
  line L602 (162.8583, 68) -> (166.6111, 61.5)
  line L603 (166.6111, 61.5) -> (162.8583, 55)
  line L604 (163.4357, 54) -> (167.1885, 60.5)
  line L605 (167.1885, 47.5) -> (163.4357, 54)
  line L606 (174.694, 47.5) -> (167.1885, 47.5)
  line L607 (178.4468, 54) -> (174.694, 47.5)
  line L608 (174.694, 60.5) -> (178.4468, 54)
  line L609 (167.1885, 60.5) -> (174.694, 60.5)
  line L610 (162.8583, 40) -> (155.3528, 40)
  line L611 (155.3528, 40) -> (151.6, 46.5)
  line L612 (151.6, 46.5) -> (155.3528, 53)
  line L613 (155.3528, 53) -> (162.8583, 53)
  line L614 (162.8583, 53) -> (166.6111, 46.5)
  line L615 (166.6111, 46.5) -> (162.8583, 40)
  line L616 (163.4357, 39) -> (167.1885, 45.5)
  line L617 (167.1885, 32.5) -> (163.4357, 39)
  line L618 (174.694, 32.5) -> (167.1885, 32.5)
  line L619 (178.4468, 39) -> (174.694, 32.5)
  line L620 (174.694, 45.5) -> (178.4468, 39)
  line L621 (167.1885, 45.5) -> (174.694, 45.5)
  line L622 (162.8583, 25) -> (155.3528, 25)
  line L623 (155.3528, 25) -> (151.6, 31.5)
  line L624 (151.6, 31.5) -> (155.3528, 38)
  line L625 (155.3528, 38) -> (162.8583, 38)
  line L626 (162.8583, 38) -> (166.6111, 31.5)
  line L627 (166.6111, 31.5) -> (162.8583, 25)
  line L628 (163.4357, 24) -> (167.1885, 30.5)
  line L629 (167.1885, 17.5) -> (163.4357, 24)
  line L630 (174.694, 17.5) -> (167.1885, 17.5)
  line L631 (178.4468, 24) -> (174.694, 17.5)
  line L632 (174.694, 30.5) -> (178.4468, 24)
  line L633 (167.1885, 30.5) -> (174.694, 30.5)
  line L634 (162.8583, 10) -> (155.3528, 10)
  line L635 (155.3528, 10) -> (151.6, 16.5)
  line L636 (151.6, 16.5) -> (155.3528, 23)
  line L637 (155.3528, 23) -> (162.8583, 23)
  line L638 (162.8583, 23) -> (166.6111, 16.5)
  line L639 (166.6111, 16.5) -> (162.8583, 10)
  point P0 (95.0422, 0)
  point P1 (17.5056, 121.5)
  point P2 (29.3412, 114)
  point P3 (36.8468, 9)
  point P4 (21.8357, 9)
  point P5 (25.5885, 15.5)
  point P6 (33.094, 15.5)
  point P7 (60.5468, 9)
  point P8 (45.5357, 9)
  point P9 (49.2885, 15.5)
  point P10 (56.794, 15.5)
  point P11 (84.2468, 9)
  point P12 (69.2357, 9)
  point P13 (72.9885, 15.5)
  point P14 (80.494, 15.5)
  point P15 (107.9468, 9)
  point P16 (92.9357, 9)
  point P17 (96.6885, 15.5)
  point P18 (104.194, 15.5)
  point P19 (131.6468, 9)
  point P20 (116.6357, 9)
  point P21 (120.3885, 15.5)
  point P22 (127.894, 15.5)
  point P23 (155.3468, 9)
  point P24 (140.3357, 9)
  point P25 (144.0885, 15.5)
  point P26 (151.594, 15.5)
  point P27 (154.7468, 114)
  point P28 (154.7468, 99)
  point P29 (154.7468, 84)
  point P30 (154.7468, 69)
  point P31 (154.7468, 54)
  point P32 (154.7468, 39)
  point P33 (154.7468, 24)
  point P34 (167.1885, 15.5)
  point P35 (174.694, 15.5)
  dimension "d16" = 13
  dimension "d17" = 3
  dimension "d19" = 3
  dimension "d22" = 23.7
  dimension "d25" = 15
  dimension "d47" = 1
  dimension "d51" = 23.1
  dimension "d134" = 2
  dimension "d135" = 1
  dimension "d136" = 1.0248
  constraints: 1274 end point, 5 parallel, 4 horizontal, 4 vertical, 1 collinear, 1 perpendicular, 1295 other
  measures "d16" distance between parallel lines of L12 L9
  measures "d17" distance from line of L6 L10.end
  measures "d19" distance between parallel lines of L7 L12
  measures "d22" distance of L9.start L21.start
  measures "d25" distance of L9.start L81.start
  measures "d47" distance between parallel lines of L85 L17
  measures "d51" distance of L63.start point (154.747, 114)
  measures "d134" distance between parallel lines of L84 L9
  measures "d135" distance between parallel lines of L18 L14
  measures "d136" distance between parallel lines of L20 L22
extrude "HonycombLongSide" [suppressed]